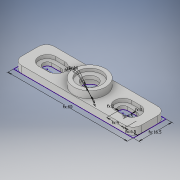
# Autodesk Inventor part: coffee
Saved by Autodesk Inventor 2017 (Build 210142000, 142)
## iProperties
Created: 2019-12-05
Part Number: coffee
Material: Generic
Document SubType Name: Modeling
Designer: Christian
Density: 1 g/cm^3
Appearance: Default
Author: Christian
Autodesk Inventor part; units mm, degrees
ref_plane "YZ Plane" through (0, 0, 0) normal (1, 0, 0) x (0, 1, 0)
ref_plane "XZ Plane" through (0, 0, 0) normal (0, 1, 0) x (-1, 0, 0)
ref_plane "XY Plane" through (0, 0, 0) normal (0, 0, 1) x (1, 0, 0)
sketch "skt_base" plane through (0, 0, 0) normal (0, 0, 1) x (1, 0, 0)
  line L0 (-30, -8.25) -> (30, -8.25)
  line L1 (30, -8.25) -> (30, 8.25)
  line L2 (30, 8.25) -> (-30, 8.25)
  line L3 (-30, 8.25) -> (-30, -8.25)
  line L4 (-30, -8.25) -> (30, 8.25) construction
  line L5 (30, -8.25) -> (-30, 8.25) construction
  line L6 (-30, 0) -> (30, 0) construction
  line L7 (0, -8.25) -> (0, 8.25) construction
  line L8 (14.5, 0) -> (23.5, 0) construction
  line L9 (16.75, -2.25) -> (21.25, -2.25)
  line L10 (21.25, 2.25) -> (16.75, 2.25)
  arc A0 (16.75, 2.25) -> (16.75, -2.25) centre (16.75, 0) ccw
  arc A1 (21.25, -2.25) -> (21.25, 2.25) centre (21.25, 0) ccw
  line L11 (12.5, 0) -> (25.5, 0) construction
  line L12 (16.75, -4.25) -> (21.25, -4.25)
  line L13 (21.25, 4.25) -> (16.75, 4.25)
  arc A2 (16.75, 4.25) -> (16.75, -4.25) centre (16.75, 0) ccw
  arc A3 (21.25, -4.25) -> (21.25, 4.25) centre (21.25, 0) ccw
  line L14 (-16.75, -2.25) -> (-21.25, -2.25)
  line L15 (-21.25, 2.25) -> (-16.75, 2.25)
  arc A4 (-16.75, -2.25) -> (-16.75, 2.25) centre (-16.75, 0) ccw
  arc A5 (-21.25, 2.25) -> (-21.25, -2.25) centre (-21.25, 0) ccw
  line L16 (-16.75, -4.25) -> (-21.25, -4.25)
  line L17 (-21.25, 4.25) -> (-16.75, 4.25)
  arc A6 (-16.75, -4.25) -> (-16.75, 4.25) centre (-16.75, 0) ccw
  arc A7 (-21.25, 4.25) -> (-21.25, -4.25) centre (-21.25, 0) ccw
  circle A8 centre (0, 0) radius 3.75
  circle A9 centre (0, 0) radius 6
  circle A10 centre (0, 0) radius 8
  point P0 (0, 0)
  point P1 (19, 0)
  point P2 (19, 0)
  point P3 (0, 0)
  dimension "d13" = 60
  dimension "d14" = 16.5
  dimension "d29" = 6.5
  dimension "d30" = 4.5
  dimension "d31" = 9
  dimension "d32" = 2
  dimension "d33" = 2
  dimension "d47" = 16
  dimension "d48" = 12
  dimension "d49" = 7.5
  constraints: 40 end point, 20 point on circle, 12 symmetric about line, 11 centre point, 10 midpoint, 8 point on line, 8 tangent, 4 coincident, 4 parallel, 1 horizontal, 1 perpendicular, 4 other
  measures "d13" distance of L0.start L0.end
  measures "d14" distance of L0.end L1.end
  measures "d29" distance of L6.end L8.end
  measures "d30" distance between parallel lines of L9 L10
  measures "d31" distance of L8.end L8.start
  measures "d32" distance between parallel lines of L13 L10
  measures "d33" distance of L11.start L8.start
  measures "d47" diameter of A10
  measures "d48" diameter of A9
  measures "d49" diameter of A8
extrude "base" add sketch "skt_base" along normal blind 3.5 contours L3 L2 L1 L0
extrude "screw_head" add sketch "skt_base" along normal blind 1.75 contours A2 L13 A3 L12 | L16 A7 L17 A6
extrude "handle_support" add sketch "skt_base" along normal blind 7 contours A10
extrude "handle_guide" add sketch "skt_base" along normal blind 5.5 contours A9
extrude "handle_screw_head" cut sketch "skt_base" along normal blind 3.7 contours A9
fillet "side_fillets" radius 4 4 edges at (-30, -8.25, 1.75) (30, -8.25, 1.75) (30, 8.25, 1.75) (-30, 8.25, 1.75)
equation "\"d13\" = base_l"
equation "\"d14\" = base_w"
equation "\"d29\" = base_screw_b"
equation "\"d30\" = base_screw_w"
equation "\"d31\" = base_screw_l"
equation "\"d32\" = base_screw_p"
equation "\"d33\" = base_screw_p"
equation "\"d47\" = handle_screw_e"
equation "\"d48\" = handle_screw_p"
equation "\"d49\" = handle_screw_d"
equation "\"d15\" = base_t"
equation "\"d34\" = base_screw_t"
equation "\"d50\" = handle_screw_h"
equation "\"d52\" = handle_screw_h - handle_screw_b"
equation "\"d54\" = handle_screw_h - 2.2 * handle_screw_b"
equation "\"wall_inner_diam\" = 2"
equation "\"wall_outer_diam\" = 1"
equation "\"wall_height\" = 8"
equation "\"leg_diam\" = 3"
equation "\"leg_height\" = 4"
equation "\"wall_widh\" = 8"
equation "\"base_screw_w\" = 4.5"
equation "\"base_t\" = 3.5"
equation "\"base_w\" = 16.5"
equation "\"base_l\" = 60"
equation "\"base_screw_p\" = 2"
equation "\"base_screw_l\" = 9"
equation "\"base_screw_t\" = 1.75"
equation "\"base_screw_b\" = 6.5"
equation "\"handle_screw_p\" = 12"
equation "\"handle_screw_d\" = 7.5"
equation "\"handle_screw_e\" = 16"
equation "\"handle_screw_b\" = 1.5"
equation "\"handle_screw_h\" = 7"
equation "\"d44\" = 7.5"
equation "\"d45\" = 16"
equation "\"d46\" = 12"
body "Solid2"
